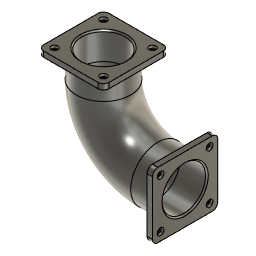
MAD 3 v1 (Autodesk Fusion 360 design; units mm, degrees)
Autodesk Fusion 360 part; units mm, degrees
sketch "Sketch1" plane through (0, 0, 0) normal (0, 1, 0) x (1, 0, 0)
  line L0 (0, -10) -> (0, -15)
  line L1 (10, 0) -> (15, 0)
  arc A0 (10, 0) -> (0, -10) centre (10, -10) ccw
  dimension "d1" = 15
  dimension "d2" = 15
  dimension "d3" = 10
  constraint vertical L0
  constraint perpendicular L0 L1
  constraint coincident origin L1
  constraint coincident origin L0
  constraint tangent L1 A0
  constraint tangent L0 A0
  measures "d1" distance of origin L0.end
  measures "d2" distance of origin L1.end
  measures "d3" radius of A0
  measures "d10" radius of L1.start
  measures "d26" radius of L1.start
pipe "Pipe1" add diameter 10 wall 1 path "Sketch1" along L0 A0 L1
sketch "Sketch2" plane through (15, 0, 0) normal (1, 0, 0) x (0, 1, 0)
  circle A0 centre (0, 0) radius 4
  circle A1 centre (0, 0) radius 5
  line L0 (5, 6) -> (-5, 6)
  line L1 (-6, 5) -> (-6, -5)
  line L2 (-5, -6) -> (5, -6)
  line L3 (6, -5) -> (6, 5)
  line L4 (6, 6) -> (-6, -6) construction
  line L5 (-6, 6) -> (6, -6) construction
  arc A2 (-6, -5) -> (-5, -6) centre (-5, -5) ccw
  arc A3 (5, -6) -> (6, -5) centre (5, -5) ccw
  arc A4 (6, 5) -> (5, 6) centre (5, 5) ccw
  arc A5 (-5, 6) -> (-6, 5) centre (-5, 5) ccw
  circle A6 centre (-4.5, 4.5) radius 0.625
  circle A7 centre (-4.5, -4.5) radius 0.625
  circle A8 centre (4.5, -4.5) radius 0.625
  circle A9 centre (4.5, 4.5) radius 0.625
  dimension "d8" = 12
  dimension "d9" = 12
  dimension "d10" = 1
  dimension "d11" = 1.25
  dimension "d12" = 1.5
  dimension "d14" = 360
  constraint horizontal L0
  constraint perpendicular L0 L1
  constraint parallel L0 L2
  constraint parallel L1 L3
  constraint coincident L4 A0.centre
  constraint coincident L5 A0.centre
  constraint coincident A0.centre A1.centre
  constraint coincident L4.end L1
  constraint coincident L4.end L2
  constraint tangent L1 A2
  constraint tangent L2 A2
  constraint coincident L5.end L2
  constraint coincident L5.end L3
  constraint tangent L2 A3
  constraint tangent L3 A3
  constraint equal A2 A3
  constraint coincident L4.start L3
  constraint coincident L4.start L0
  constraint tangent L3 A4
  constraint tangent L0 A4
  constraint equal A2 A4
  constraint coincident L5.start L0
  constraint coincident L5.start L1
  constraint tangent L0 A5
  constraint tangent L1 A5
  constraint equal A2 A5
  constraint coincident L5 A6.centre
  measures "d8" distance of L4.end L5.end
  measures "d9" distance of L5.start L4.end
  measures "d10" radius of A2
  measures "d11" diameter of A6
  measures "d12" distance of L1 A6.centre
extrude "Extrude1" add sketch "Sketch2" against normal blind 1 contours L0 L1 L2 L3 A2 A3 A4 A5 | A6 | A7 | A8 | A9
extrude "Extrude2" cut sketch "Sketch2" against normal blind 0.5 contours A6 | A7 | A8 | A9
hole "Hole1" at (14.5, -4.5, 4.5) direction (-1, 0, 0) diameter 0.75 depth 1 tip angle 180
pattern_circular "C-Pattern1" count 4 over 360 about axis through (15, 0, 0) along (-1, 0, 0) of "Hole1"
sketch "Sketch3" plane through (0, 0, 15) normal (0, 0, 1) x (-1, 0, 0)
  circle A0 centre (0, 0) radius 4
  circle A1 centre (0, 0) radius 5
  line L0 (-5, 6) -> (5, 6)
  line L1 (6, 5) -> (6, -5)
  line L2 (5, -6) -> (-5, -6)
  line L3 (-6, -5) -> (-6, 5)
  line L4 (-6, 6) -> (6, -6) construction
  line L5 (6, 6) -> (-6, -6) construction
  arc A2 (5, -6) -> (6, -5) centre (5, -5) ccw
  arc A3 (-6, -5) -> (-5, -6) centre (-5, -5) ccw
  arc A4 (-5, 6) -> (-6, 5) centre (-5, 5) ccw
  arc A5 (6, 5) -> (5, 6) centre (5, 5) ccw
  circle A6 centre (4.5, -4.5) radius 0.625
  circle A7 centre (4.5, 4.5) radius 0.625
  circle A8 centre (-4.5, 4.5) radius 0.625
  circle A9 centre (-4.5, -4.5) radius 0.625
  dimension "d24" = 12
  dimension "d25" = 12
  dimension "d26" = 1
  dimension "d27" = 1.25
  dimension "d28" = 1.5
  dimension "d30" = 360
  constraint horizontal L0
  constraint perpendicular L0 L1
  constraint parallel L0 L2
  constraint parallel L1 L3
  constraint coincident L4 A0.centre
  constraint coincident L5 A0.centre
  constraint coincident A0.centre A1.centre
  constraint coincident L4.end L1
  constraint coincident L4.end L2
  constraint tangent L1 A2
  constraint tangent L2 A2
  constraint coincident L5.end L2
  constraint coincident L5.end L3
  constraint tangent L2 A3
  constraint tangent L3 A3
  constraint equal A2 A3
  constraint coincident L4.start L3
  constraint coincident L4.start L0
  constraint tangent L3 A4
  constraint tangent L0 A4
  constraint equal A2 A4
  constraint coincident L5.start L0
  constraint coincident L5.start L1
  constraint tangent L0 A5
  constraint tangent L1 A5
  constraint equal A2 A5
  constraint coincident L4 A6.centre
  measures "d24" distance of L4.end L5.end
  measures "d25" distance of L5.start L4.end
  measures "d26" radius of A2
  measures "d27" diameter of A6
  measures "d28" distance of L1 A6.centre
extrude "Extrude3" add sketch "Sketch3" against normal blind 1 contours L0 L1 L2 L3 A2 A3 A4 A5 | A6 | A7 | A8 | A9
extrude "Extrude4" cut sketch "Sketch3" against normal blind 0.5 contours A6 | A7 | A8 | A9
hole "Hole2" at (-4.5, 4.5, 14.5) direction (0, 0, -1) diameter 0.75 depth 1 tip angle 180
pattern_circular "C-Pattern2" count 4 over 360 about axis through (0, 0, 15) along (0, 0, -1) of "Hole2"
chamfer "Chamfer1" distance 0.25 angle 45 2 edges at (3.7293, -1.4465, 15) (15, 1.4465, 3.7293)
